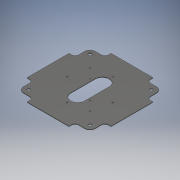
# Autodesk Inventor part: -ZPanel_PCB
Saved by Autodesk Inventor 2018 (Build 220112000, 112)
## iProperties
Created: 2018-11-03
Part Number: -ZPanel_PCB
Material: Epoxy Resin
Document SubType Name: Modeling
Designer: Bradley
Density: 1.14 g/cm^3
Appearance: Smooth - Dark Gray
Mass: 5.79181 g
Surface Area: 172.339 cm^2
Volume: 5.08053 cm^3
Author: Bradley
Autodesk Inventor part; units mm, degrees
ref_plane "YZ Plane" through (0, 0, 0) normal (1, 0, 0) x (0, 1, 0)
ref_plane "XZ Plane" through (0, 0, 0) normal (0, 1, 0) x (-1, 0, 0)
ref_plane "XY Plane" through (0, 0, 0) normal (0, 0, 1) x (1, 0, 0)
sketch "Sketch1" plane through (0, 0, 0) normal (0, 0, 1) x (1, 0, 0)
  line L0 (-48, -48) -> (48, -48)
  line L1 (48, -48) -> (48, 48)
  line L2 (48, 48) -> (-48, 48)
  line L3 (-48, 48) -> (-48, -48)
  line L4 (-48, -48) -> (48, 48) construction
  line L5 (48, -48) -> (-48, 48) construction
  circle A0 centre (0, 0) radius 40 construction
  circle A1 centre (0, 0) radius 8
  line L6 (-45, -32.5) -> (45, -32.5) construction
  line L7 (45, -32.5) -> (45, 32.5) construction
  line L8 (45, 32.5) -> (-45, 32.5) construction
  line L9 (-45, 32.5) -> (-45, -32.5) construction
  line L10 (-45, -32.5) -> (45, 32.5) construction
  line L11 (45, -32.5) -> (-45, 32.5) construction
  line L12 (-28, -46.5) -> (28, -46.5) construction
  line L13 (28, -46.5) -> (28, 46.5) construction
  line L14 (28, 46.5) -> (-28, 46.5) construction
  line L15 (-28, 46.5) -> (-28, -46.5) construction
  line L16 (-28, -46.5) -> (28, 46.5) construction
  line L17 (28, -46.5) -> (-28, 46.5) construction
  circle A2 centre (-45, 32.5) radius 4 construction
  circle A3 centre (-28, 46.5) radius 4 construction
  line L18 (-35, -35) -> (35, -35) construction
  line L19 (35, -35) -> (35, 35) construction
  line L20 (35, 35) -> (-35, 35) construction
  line L21 (-35, 35) -> (-35, -35) construction
  line L22 (-35, -35) -> (35, 35) construction
  line L23 (35, -35) -> (-35, 35) construction
  circle A4 centre (-35, 35) radius 3 construction
  line L24 (-24, 48) -> (-24, 45)
  arc A5 (-28, 41) -> (-24, 45) centre (-28, 45) ccw
  line L25 (-28, 41) -> (-35, 41)
  arc A6 (-35, 41) -> (-41, 35) centre (-35, 35) ccw
  line L26 (-41, 35) -> (-41, 28)
  arc A7 (-45, 24) -> (-41, 28) centre (-45, 28) ccw
  line L27 (-45, 24) -> (-48, 24)
  line L28 (48, 24) -> (45, 24)
  arc A8 (41, 28) -> (45, 24) centre (45, 28) ccw
  line L29 (41, 28) -> (41, 35)
  arc A9 (41, 35) -> (35, 41) centre (35, 35) ccw
  line L30 (35, 41) -> (28, 41)
  arc A10 (24, 45) -> (28, 41) centre (28, 45) ccw
  line L31 (24, 45) -> (24, 48)
  line L32 (48, -24) -> (45, -24)
  arc A11 (45, -24) -> (41, -28) centre (45, -28) ccw
  line L33 (41, -28) -> (41, -35)
  arc A12 (35, -41) -> (41, -35) centre (35, -35) ccw
  line L34 (35, -41) -> (28, -41)
  arc A13 (28, -41) -> (24, -45) centre (28, -45) ccw
  line L35 (24, -45) -> (24, -48)
  line L36 (-24, -48) -> (-24, -45)
  arc A14 (-24, -45) -> (-28, -41) centre (-28, -45) ccw
  line L37 (-28, -41) -> (-35, -41)
  arc A15 (-41, -35) -> (-35, -41) centre (-35, -35) ccw
  line L38 (-41, -35) -> (-41, -28)
  arc A16 (-41, -28) -> (-45, -24) centre (-45, -28) ccw
  line L39 (-45, -24) -> (-48, -24)
  line L40 (0, 14) -> (0, -14) construction
  line L41 (8, 14) -> (8, -14)
  line L42 (-8, -14) -> (-8, 14)
  arc A17 (8, 14) -> (-8, 14) centre (0, 14) ccw
  arc A18 (-8, -14) -> (8, -14) centre (0, -14) ccw
  point P0 (-7.746, 2)
  point P1 (-7.746, -2)
  dimension "d0" = 96
  dimension "d1" = 96
  dimension "d3" = 80
  dimension "d7" = 16
  dimension "d48" = 90
  dimension "d49" = 65
  dimension "d50" = 56
  dimension "d51" = 93
  dimension "d52" = 8
  dimension "d53" = 70
  dimension "d54" = 6
  dimension "d55" = 24
  dimension "d56" = 24
  dimension "d57" = 4
  dimension "d58" = 41
  dimension "d59" = 28
  constraints: 88 end point, 30 point on circle, 28 tangent, 19 centre point, 18 perpendicular, 11 equal radius, 11 point on line, 9 midpoint, 9 parallel, 7 collinear, 5 coincident, 5 horizontal, 4 equal length, 2 vertical, 1 concentric
  measures "d0" distance of L2.end L1.end
  measures "d1" distance of L1.end L0.end
  measures "d3" diameter of A0
  measures "d7" diameter of A1
  measures "d48" distance of L8.end L7.end
  measures "d49" distance of L7.end L6.end
  measures "d50" distance of L14.end L13.end
  measures "d51" distance of L13.end L12.end
  measures "d52" diameter of A2
  measures "d53" distance of L20.end L19.end
  measures "d54" diameter of A4
  measures "d55" distance from line of point (0, 0) L24
  measures "d56" distance from line of point (0, 0) L27
  measures "d57" radius of A5
  measures "d58" distance from line of point (0, 0) L26
  measures "d59" distance of L41.start L41.end
extrude "Extrusion1" add sketch "Sketch1" along normal mid plane 0.6 contours L36 A14 L37 A15 L38 A16 L39 L3 L27 A7 L26 A6 L25 A5 L24 L2 L31 A10 L30 A9 L29 A8 L28 L1 L32 A11 L33 A12 L34 A13 L35 L0
fillet "Fillet1" radius 0.5 8 edges at (-24, -48, 0) (-48, -24, 0) (-48, 24, 0) (-24, 48, 0) (24, 48, 0) (48, 24, 0) (48, -24, 0) (24, -48, 0)
sketch "Sketch2" plane through (0, 0, 0.3) normal (0, 0, 1) x (1, 0, 0)
  line L0 (21.2132, -21.2132) -> (10.6066, -10.6066) construction
  line L1 (-21.2132, 21.2132) -> (-10.6066, 10.6066) construction
  line L2 (-23.5, -48) -> (23.5, -48) projected
  line L3 (48, -23.5) -> (48, 23.5) projected
  line L4 (23.5, 48) -> (-23.5, 48) projected
  line L5 (-48, 23.5) -> (-48, -23.5) projected
  circle A0 centre (0, 0) radius 15 construction
  line L6 (-24, 47.5) -> (-24, 45) projected
  arc A1 (-28, 41) -> (-24, 45) centre (-28, 45) ccw projected
  line L7 (-28, 41) -> (-35, 41) projected
  arc A2 (-35, 41) -> (-41, 35) centre (-35, 35) ccw projected
  line L8 (-41, 35) -> (-41, 28) projected
  arc A3 (-45, 24) -> (-41, 28) centre (-45, 28) ccw projected
  line L9 (-45, 24) -> (-47.5, 24) projected
  line L10 (-47.5, -24) -> (-45, -24) projected
  arc A4 (-41, -28) -> (-45, -24) centre (-45, -28) ccw projected
  line L11 (-41, -28) -> (-41, -35) projected
  arc A5 (-41, -35) -> (-35, -41) centre (-35, -35) ccw projected
  line L12 (-35, -41) -> (-28, -41) projected
  arc A6 (-24, -45) -> (-28, -41) centre (-28, -45) ccw projected
  line L13 (-24, -45) -> (-24, -47.5) projected
  line L14 (24, -47.5) -> (24, -45) projected
  arc A7 (28, -41) -> (24, -45) centre (28, -45) ccw projected
  line L15 (28, -41) -> (35, -41) projected
  arc A8 (35, -41) -> (41, -35) centre (35, -35) ccw projected
  line L16 (41, -35) -> (41, -28) projected
  arc A9 (45, -24) -> (41, -28) centre (45, -28) ccw projected
  line L17 (45, -24) -> (47.5, -24) projected
  line L18 (47.5, 24) -> (45, 24) projected
  arc A10 (41, 28) -> (45, 24) centre (45, 28) ccw projected
  line L19 (41, 28) -> (41, 35) projected
  arc A11 (41, 35) -> (35, 41) centre (35, 35) ccw projected
  line L20 (35, 41) -> (28, 41) projected
  arc A12 (24, 45) -> (28, 41) centre (28, 45) ccw projected
  line L21 (24, 45) -> (24, 47.5) projected
  arc A13 (23.5, -48) -> (24, -47.5) centre (23.5, -47.5) ccw projected
  arc A14 (47.5, -24) -> (48, -23.5) centre (47.5, -23.5) ccw projected
  arc A15 (48, 23.5) -> (47.5, 24) centre (47.5, 23.5) ccw projected
  arc A16 (24, 47.5) -> (23.5, 48) centre (23.5, 47.5) ccw projected
  arc A17 (-23.5, 48) -> (-24, 47.5) centre (-23.5, 47.5) ccw projected
  arc A18 (-47.5, 24) -> (-48, 23.5) centre (-47.5, 23.5) ccw projected
  arc A19 (-48, -23.5) -> (-47.5, -24) centre (-47.5, -23.5) ccw projected
  arc A20 (-24, -47.5) -> (-23.5, -48) centre (-23.5, -47.5) ccw projected
  line L22 (-8, -14) -> (-8, 14) projected
  arc A21 (8, 14) -> (-8, 14) centre (0, 14) ccw projected
  line L23 (8, 14) -> (8, -14) projected
  arc A22 (-8, -14) -> (8, -14) centre (0, -14) ccw projected
  dimension "d12" = 15
  dimension "d33" = 135
  dimension "d34" = 30
  constraints: 5 coincident, 4 end point, 2 collinear, 2 point on circle, 1 centre point, 1 point on line
  measures "d12" distance of L1.start L1.end
  measures "d33" angle of L2 L1
  measures "d34" diameter of A0
hole "Hole1" at (-10.6066, 10.6066, 0.3) at (-21.2132, 21.2132, 0.3) at (10.6066, -10.6066, 0.3) at (21.2132, -21.2132, 0.3) direction (0, 0, -1) diameter 1 end through all
sketch "Sketch3" plane through (0, 0, 0.3) normal (0, 0, 1) x (1, 0, 0)
  point P0 (0, 0)
  point P1 (-26, 0)
  point P2 (0, -26)
  point P3 (26, 0)
  point P4 (0, 26)
  dimension "d21" = 26
  dimension "d24" = 360
  constraints: 1 horizontal alignment, 5 other
  measures "d21" distance of point (-26, 0) point (0, 0)
hole "Hole2" at (-26, 0, 0.3) at (0, -26, 0.3) at (26, 0, 0.3) at (0, 26, 0.3) direction (0, 0, -1) diameter 1.6 end through all
sketch "Sketch4" plane through (0, 0, 0.3) normal (0, 0, 1) x (1, 0, 0)
  line L0 (-35, -35) -> (35, -35) construction
  line L1 (35, -35) -> (35, 35) construction
  line L2 (35, 35) -> (-35, 35) construction
  line L3 (-35, 35) -> (-35, -35) construction
  line L4 (-35, -35) -> (35, 35) construction
  line L5 (35, -35) -> (-35, 35) construction
  point P0 (0, 0)
  dimension "d35" = 70
  constraints: 12 end point, 4 coincident, 2 midpoint, 2 parallel, 2 perpendicular, 1 horizontal
  measures "d35" distance of L2.end L1.end
hole "Hole3" at (-35, 35, 0.3) at (35, 35, 0.3) at (35, -35, 0.3) at (-35, -35, 0.3) direction (0, 0, -1) diameter 3.4 end through all clearance for "Flat Head Machine Screw" size "M3" standard "Ansi Metric M Profile"
equation "\"d56\" = d55"
body "Solid1"
